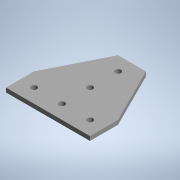
# Autodesk Inventor part: 40-4340
Saved by Autodesk Inventor 2021 (Build 250183000, 183)
## iProperties
Part Number: 40-4340
Material: Generic
Catalog Web Link: www.cadenas.de
Description: 25-4140, 25-4140-Black, 30-4340, 30-4340-Black, 40-4340, 40-4340-Black, 45-4340, 45-4340-Black-5 Hole Tee Joining Plate
Vendor: 8020
Document SubType Name: Modeling
Designer: partserver
Manufacturer: 8020
Mass: 65.5651 g
Surface Area: 251.534 cm^2
Volume: 65.5651 cm^3
Density: 1 g/cm^3
Appearance: PSOLRGB-191-191-191
Category: PARTsolutions
Company: 8020
PSOL_IDENT_0: {$CADENAS_DATA\23d-libs\8020\metric\joining_plates\25_4140.prj},242 {VTYP=3D},{NB=40-4340},{LINA=40-
PSOL_IDENT_1: 4340},{NN=25-4140, 25-4140-Black, 30-4340, 30-4340-Black, 40-4340, 40-4340-Black, 45-4340, 45-4340-B
PSOL_IDENT_2: lack},{DATE=31.07.2020 09:21:28},{GEOMDATE=16.01.2019 16:29:06},{VERSION=},{LINEID=30},{WBVAR=},{WBN
PSOL_IDENT_3: UMERIC=}  {NB=40-4340},{LINA=40-4340},{KT=DUMMY},{PN=40-4340},{A=120.00},{B=40.00},{C=6.00},{D=8.33}
PSOL_IDENT_4: ,{E=20.00},{F=40.00},{W=.168},{A1=20.0000},{C1=60.000},{C2=20.000},{C3=100.000},{D1=6.000},{COLOR=.7
PSOL_IDENT_5: 5,.75,.75}
NB: 40-4340
NN: 25-4140, 25-4140-Black, 30-4340, 30-4340-Black, 40-4340, 40-4340-Black, 45-4340, 45-4340-Black
NT: 5 Hole Tee Joining Plate
NBSYN: $PN.
LINA: 40-4340
CATALOG: 80/20
PN: 40-4340
A: 120
B: 40
C: 6
D: 8.33
E: 20
F: 40
W: .168
SUPPLIER: 8020
ARTICLENO: 40-4340
BOMINFO: 40-4340
CREATOR: CADENAS GmbH
Title: 40-4340
Author: Cadenas PARTsolutions
Comments: 5 Hole Tee Joining Plate
Autodesk Inventor part; units mm, degrees
ref_plane "YZ Plane" through (0, 0, 0) normal (1, 0, 0) x (0, 1, 0)
ref_plane "XZ Plane" through (0, 0, 0) normal (0, 1, 0) x (-1, 0, 0)
ref_plane "XY Plane" through (0, 0, 0) normal (0, 0, 1) x (1, 0, 0)
sketch "Sketch_1" plane through (0, 0, 0) normal (0, 0, 1) x (1, 0, 0)
  line L0 (-60, 40) -> (-60, 0)
  line L1 (-60, 0) -> (60, 0)
  line L2 (60, 0) -> (60, 40)
  line L3 (60, 40) -> (20, 120)
  line L4 (20, 120) -> (-20, 120)
  line L5 (-20, 120) -> (-60, 40)
  circle A0 centre (40, 20) radius 4.165
  circle A1 centre (0, 60) radius 4.165
  circle A2 centre (0, 100) radius 4.165
  circle A3 centre (0, 20) radius 4.165
  circle A4 centre (-40, 20) radius 4.165
  constraints: 12 end point, 5 centre point
extrude "Extrusion1" add sketch "Sketch_1" along normal blind 6
body "Solid1"
